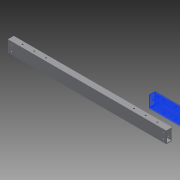
# Autodesk Inventor part: Component 1
Saved by Autodesk Inventor 2015 (Build 190159000, 159)
## iProperties
Created: 2015-01-14
Part Number: Component 1
Material: Generic
Document SubType Name: Modeling
Designer: chapale16
Density: 1 g/cm^3
Appearance: Default
Author: chapale16
Autodesk Inventor part; units mm, degrees
ref_plane "YZ Plane" through (0, 0, 0) normal (1, 0, 0) x (0, 1, 0)
ref_plane "XZ Plane" through (0, 0, 0) normal (0, 1, 0) x (-1, 0, 0)
ref_plane "XY Plane" through (0, 0, 0) normal (0, 0, 1) x (1, 0, 0)
sketch "Sketch1" plane through (0, 0, 0) normal (0, 0, 1) x (1, 0, 0)
  line L0 (0, 0) -> (-685.8, 0)
  line L1 (-685.8, 0) -> (-685.8, 50.8)
  line L2 (-685.8, 50.8) -> (0, 50.8)
  line L3 (0, 50.8) -> (0, 0)
  dimension "d0" = 50.8
  dimension "d1" = 685.8
  constraints: 8 end point, 2 parallel, 1 horizontal, 1 perpendicular
  measures "d0" distance of L2.end L0.start
  measures "d1" distance between parallel lines of L3 L1
extrude "Extrusion1" add sketch "Sketch1" along normal blind 25.4
sketch "Sketch2" plane through (0, 0, 0) normal (1, 0, 0) x (0, 0, -1)
  line L0 (-22.225, 47.625) -> (-3.175, 47.625)
  line L1 (-3.175, 47.625) -> (-3.175, 3.175)
  line L2 (-3.175, 3.175) -> (-22.225, 3.175)
  line L3 (-22.225, 3.175) -> (-22.225, 47.625)
  line L4 (0, 50.8) -> (0, 0) projected
  line L5 (0, 50.8) -> (-25.4, 50.8) projected
  line L6 (-25.4, 50.8) -> (-25.4, 0)
  line L7 (-25.4, 0) -> (0, 0)
  dimension "d5" = 3.175
  dimension "d6" = 3.175
  dimension "d7" = 3.175
  dimension "d8" = 3.175
  constraints: 12 end point, 2 parallel, 2 perpendicular, 1 horizontal, 1 vertical
  measures "d5" distance between parallel lines of L4 L1
  measures "d6" distance between parallel lines of L5 L0
  measures "d7" distance between parallel lines of L6 L3
  measures "d8" distance between parallel lines of L7 L2
extrude "Extrusion2" cut sketch "Sketch2" against normal blind 685.8 contours L0 L1 L2 L3
fillet "Fillet1" radius 3.175 1 edges at (0, 25.4, 0)
fillet "Fillet2" radius 3.175 1 edges at (-685.8, 25.4, 0)
sketch "Sketch3" plane through (-685.8, 0, 25.4) normal (0, -1, 0) x (1, 0, 0)
  circle A0 centre (584.2, 38.1) radius 3.175 projected
  circle A1 centre (584.2, 12.7) radius 3.175 projected
  circle A2 centre (533.4, -12.7) radius 3.175 projected
  circle A3 centre (558.8, -12.7) radius 3.175 projected
  circle A4 centre (609.6, -12.7) radius 3.175 projected
  circle A5 centre (635, -12.7) radius 3.175 projected
  circle A6 centre (584.2, -12.7) radius 3.175 projected
  line L0 (528.6375, -23.8125) -> (525.4625, -20.6375) projected
  line L1 (639.7625, -23.8125) -> (528.6375, -23.8125) projected
  line L2 (642.9375, -20.6375) -> (639.7625, -23.8125) projected
  line L3 (642.9375, -4.7625) -> (642.9375, -20.6375) projected
  line L4 (639.7625, -1.5875) -> (642.9375, -4.7625) projected
  line L5 (620.7125, -1.5875) -> (639.7625, -1.5875) projected
  arc A7 (595.3125, 23.8125) -> (620.7125, -1.5875) centre (620.7125, 23.8125) ccw projected
  line L6 (595.3125, 42.8625) -> (595.3125, 23.8125) projected
  line L7 (592.1375, 46.0375) -> (595.3125, 42.8625) projected
  line L8 (576.2625, 46.0375) -> (592.1375, 46.0375) projected
  line L9 (573.0875, 42.8625) -> (576.2625, 46.0375) projected
  line L10 (573.0875, 23.8125) -> (573.0875, 42.8625) projected
  arc A8 (547.6875, -1.5875) -> (573.0875, 23.8125) centre (547.6875, 23.8125) ccw projected
  line L11 (528.6375, -1.5875) -> (547.6875, -1.5875) projected
  line L12 (525.4625, -4.7625) -> (528.6375, -1.5875) projected
  line L13 (525.4625, -20.6375) -> (525.4625, -4.7625) projected
  circle A9 centre (101.6, 38.1) radius 3.175 projected
  circle A10 centre (101.6, 12.7) radius 3.175 projected
  circle A11 centre (152.4, -12.7) radius 3.175 projected
  circle A12 centre (127, -12.7) radius 3.175 projected
  circle A13 centre (76.2, -12.7) radius 3.175 projected
  circle A14 centre (50.8, -12.7) radius 3.175 projected
  circle A15 centre (101.6, -12.7) radius 3.175 projected
  line L14 (157.1625, -23.8125) -> (160.3375, -20.6375) projected
  line L15 (160.3375, -20.6375) -> (160.3375, -4.7625) projected
  line L16 (160.3375, -4.7625) -> (157.1625, -1.5875) projected
  line L17 (157.1625, -1.5875) -> (138.1125, -1.5875) projected
  arc A16 (112.7125, 23.8125) -> (138.1125, -1.5875) centre (138.1125, 23.8125) ccw projected
  line L18 (112.7125, 23.8125) -> (112.7125, 42.8625) projected
  line L19 (112.7125, 42.8625) -> (109.5375, 46.0375) projected
  line L20 (109.5375, 46.0375) -> (93.6625, 46.0375) projected
  line L21 (93.6625, 46.0375) -> (90.4875, 42.8625) projected
  line L22 (90.4875, 42.8625) -> (90.4875, 23.8125) projected
  arc A17 (65.0875, -1.5875) -> (90.4875, 23.8125) centre (65.0875, 23.8125) ccw projected
  line L23 (65.0875, -1.5875) -> (46.0375, -1.5875) projected
  line L24 (46.0375, -1.5875) -> (42.8625, -4.7625) projected
  line L25 (42.8625, -4.7625) -> (42.8625, -20.6375) projected
  line L26 (42.8625, -20.6375) -> (46.0375, -23.8125) projected
  line L27 (46.0375, -23.8125) -> (157.1625, -23.8125) projected
  point P0 (685.8, -25.4)
extrude "Extrusion3" cut sketch "Sketch3" against normal blind 50.8 contours A2 | A5 | A6 | A11 | A14 | A15
sketch "Sketch4" plane through (0, 0, 0) normal (0, 0, -1) x (-1, 0, 0)
  circle A0 centre (13.97, 38.1) radius 3.175 projected
  circle A1 centre (13.97, 12.7) radius 3.175 projected
  line L0 (2.54, 50.8) -> (2.54, 0) projected
  line L1 (25.4, 0) -> (2.54, 0) projected
  line L2 (25.4, 50.8) -> (25.4, 0) projected
  line L3 (2.54, 50.8) -> (25.4, 50.8) projected
  circle A2 centre (671.83, 38.1) radius 3.175 projected
  circle A3 centre (671.83, 12.7) radius 3.175 projected
  line L4 (683.26, 0) -> (683.26, 50.8) projected
  line L5 (660.4, 50.8) -> (683.26, 50.8) projected
  line L6 (660.4, 0) -> (660.4, 50.8) projected
  line L7 (683.26, 0) -> (660.4, 0) projected
  point P0 (0, 0)
extrude "Extrusion4" cut sketch "Sketch4" against normal blind 25.4 contours A0 | A1 | A2 | A3
body "Solid1"
